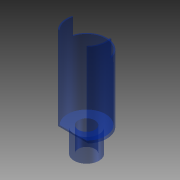
# Autodesk Inventor part: ss_inner_guide
Saved by Autodesk Inventor 2011 SP2 (Build 150309200, 309)
## iProperties
Created: 2012-05-22
Part Number: ss_inner_guide
Document SubType Name: Modeling
Designer: sungwook
Density: 1 g/cm^3
Author: sungwook
Autodesk Inventor part; units mm, degrees
ref_plane "YZ Plane" through (0, 0, 0) normal (1, 0, 0) x (0, 1, 0)
sketch "Sketch1" plane through (0, 0, 0) normal (0, 0, 1) x (1, 0, 0)
  circle A0 centre (0, 0) radius 12.25
  circle A1 centre (0, 0) radius 11.5
  dimension "d0" = 24.5
  dimension "d1" = 23
  constraints: 2 centre point, 2 coincident
  measures "d0" diameter of A0
  measures "d1" diameter of A1
extrude "Extrusion1" add sketch "Sketch1" along normal blind 49.5
sketch "Sketch2" plane through (0, 0, 49.5) normal (0, 0, 1) x (1, 0, 0)
  line L0 (-17.15, 0) -> (17.15, 0) projected
  line L1 (0, -17.15) -> (0, 17.15) projected
  line L2 (0, 0) -> (-11.8326, 3.1705)
  line L3 (0, 0) -> (-8.6621, -8.6621)
  line L4 (0, 0) -> (11.8326, 3.1705)
  line L5 (0, 0) -> (8.6621, -8.6621)
  arc A0 (11.8326, 3.1705) -> (-11.8326, 3.1705) centre (0, 0) ccw
  arc A1 (-8.6621, -8.6621) -> (8.6621, -8.6621) centre (0, 0) ccw
  dimension "d4" = 15
  dimension "d5" = 45
  constraints: 8 end point, 4 point on circle, 2 centre point, 2 coincident, 2 symmetric about line
  measures "d4" angle of L0 L2
  measures "d5" angle of L3 L0
extrude "Extrusion2" cut sketch "Sketch2" against normal blind 10
sketch "Sketch3" plane through (0, 0, 0) normal (0, 0, -1) x (-1, 0, 0)
  circle A0 centre (0, 0) radius 12.25 projected
extrude "Extrusion3" add sketch "Sketch3" along normal blind 1
sketch "Sketch4" plane through (0, 0, -1) normal (0, 0, -1) x (-1, 0, 0)
  circle A0 centre (0, 0) radius 12.25 projected
hole "Hole1" at (0, 0, -1) direction (0, 0, 1) diameter 10 end through all
ref_plane "Work Plane1" through (0, -12.25, 0) normal (0, 1, 0) x (-1, 0, 0)
sketch "Sketch5" plane through (0, -12.25, 0) normal (0, 1, 0) x (-1, 0, 0)
  line L0 (12.25, -1) -> (-12.25, -1) projected
  line L1 (11.5, 0) -> (-11.5, 0) projected
  line L2 (-5, 0) -> (-5, -1) projected
  line L3 (5, 0) -> (5, -1) projected
  line L4 (12.25, -1) -> (12.25, 49.5) projected
  line L5 (-12.25, -1) -> (-12.25, 49.5) projected
  line L6 (12.25, -1) -> (-12.25, -1) projected
  line L7 (11.8326, 49.5) -> (11.8326, 39.5) projected
  line L8 (11.8326, 39.5) -> (-11.8326, 39.5) projected
  line L9 (-11.8326, 39.5) -> (-11.8326, 49.5) projected
  line L10 (-11.8326, 49.5) -> (-8.6621, 49.5) projected
  line L11 (-8.6621, 49.5) -> (-8.6621, 39.5) projected
  line L12 (-8.6621, 39.5) -> (8.6621, 39.5) projected
  line L13 (8.6621, 39.5) -> (8.6621, 49.5) projected
  line L14 (8.6621, 49.5) -> (11.8326, 49.5) projected
  line L15 (11.5, 0) -> (11.5, 49.5) projected
  line L16 (0, -13.4846) -> (0, 73.9076) projected
  line L17 (7.5, 49) -> (-7.5, 49)
  line L18 (-7.5, 49) -> (-7.5, -1)
  line L19 (-7.5, -1) -> (7.5, -1)
  line L20 (7.5, -1) -> (7.5, 49)
  point P0 (0, 0)
  point P1 (0, 49)
  point P2 (0, 0)
  dimension "d17" = 15
  dimension "d18" = 50
  constraints: 8 end point, 2 midpoint, 2 parallel, 1 horizontal, 1 perpendicular, 1 point on line, 1 vertical alignment
  measures "d17" distance of L17.end L17.start
  measures "d18" distance of L19.end L17.start
extrude "Extrusion4" [suppressed]
ref_plane "Work Plane2" through (0, -12.25, 0) normal (0, 1, 0) x (-1, 0, 0)
sketch "Sketch8" plane through (0, 0, -1) normal (0, 0, -1) x (-1, 0, 0)
  circle A0 centre (0, 0) radius 5 projected
  circle A1 centre (0, 0) radius 7.5
  dimension "d26" = 15
  constraints: 1 centre point, 1 coincident
  measures "d26" diameter of A1
extrude "Extrusion7" add sketch "Sketch8" along normal blind 13.923
sketch "Sketch7" plane through (0, 0, 49.5) normal (0, 0, 1) x (1, 0, 0)
  arc A0 (8.6621, -8.6621) -> (11.8326, 3.1705) centre (0, 0) ccw projected
  arc A1 (8.1317, -8.1317) -> (11.1081, 2.9764) centre (0, 0) ccw projected
  line L0 (8.1317, -8.1317) -> (8.6621, -8.6621) projected
  line L1 (-10.4211, -8.1317) -> (11.1081, -8.1317)
  line L2 (11.1081, -8.1317) -> (11.1081, -13.0652)
  line L3 (11.1081, -13.0652) -> (-10.4211, -13.0652)
  line L4 (-10.4211, -13.0652) -> (-10.4211, -8.1317)
  constraints: 8 end point, 2 parallel, 1 horizontal, 1 perpendicular
extrude "Extrusion6" cut sketch "Sketch7" against normal through all
body "Solid1"
